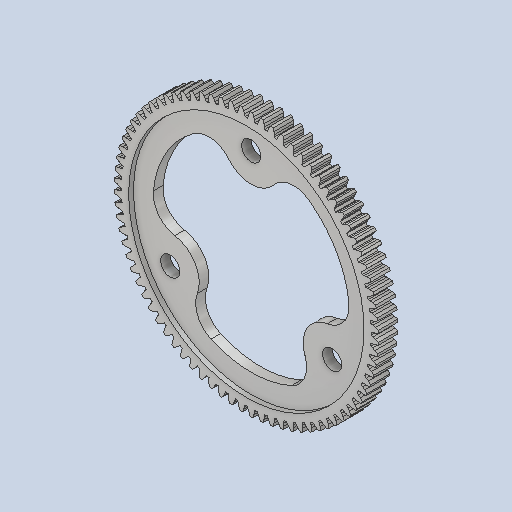
# Autodesk Inventor part: m0.5 80 初段改善
Saved by Autodesk Inventor 2022 (Build 260153000, 153)
## iProperties
Part Number: m0.5 80 初段改善
Material: アセタール樹脂、白
Document SubType Name: Modeling
Designer: user
Density: 1.425 g/cm^3
Appearance: アルミニウム - つや出し
Mass: 1.78935 g
Surface Area: 23.8506 cm^2
Volume: 1.25569 cm^3
Author: user
Autodesk Inventor part; units mm, degrees
(part 1 of 2)
ref_plane "YZ Plane" through (0, 0, 0) normal (1, 0, 0) x (0, 1, 0)
ref_plane "XZ Plane" through (0, 0, 0) normal (0, 1, 0) x (-1, 0, 0)
sketch "スケッチ3" plane through (0, 0, 0) normal (0, 0, 1) x (1, 0, 0)
  circle A0 centre (0, 0) radius 17.5
  circle A1 centre (0, 0) radius 15 construction
  circle A2 centre (-0.0185, 15) radius 3 construction
  arc A3 (1.3802, 16.4422) -> (-1.3922, 16.4412) centre (0, 0) ccw
  arc A4 (15.2271, 6.3549) -> (1.3802, 16.4422) centre (0, 0) ccw
  arc A5 (-1.3922, 16.4412) -> (-15.5317, 5.5691) centre (0, 0) ccw
  arc A6 (-15.7143, -5.031) -> (-7.6771, -14.6052) centre (0, 0) ccw
  arc A7 (-7.6771, -14.6052) -> (3.9215, -16.0272) centre (0, 0) ccw
  arc A8 (3.9215, -16.0272) -> (14.9167, -7.0527) centre (0, 0) ccw
  arc A9 (-15.5317, 5.5691) -> (-15.7143, -5.031) centre (0, 0) ccw
  arc A10 (14.9167, -7.0527) -> (15.2271, 6.3549) centre (0, 0) ccw
  circle A11 centre (-0.0185, 15) radius 1.5
  circle A12 centre (-6.525, 13.5065) radius 1.5
  circle A13 centre (-6.525, 13.5065) radius 3 construction
  circle A14 centre (-11.739, 9.3378) radius 1.5
  circle A15 centre (-11.739, 9.3378) radius 3 construction
  circle A16 centre (-14.628, 3.3197) radius 1.5
  circle A17 centre (-14.628, 3.3197) radius 3 construction
  circle A18 centre (-14.6198, -3.3559) radius 1.5
  circle A19 centre (-14.6198, -3.3559) radius 3 construction
  circle A20 centre (-11.7159, -9.3668) radius 1.5
  circle A21 centre (-11.7159, -9.3668) radius 3 construction
  circle A22 centre (-6.4915, -13.5226) radius 1.5
  circle A23 centre (-6.4915, -13.5226) radius 3 construction
  circle A24 centre (0.0185, -15) radius 1.5
  circle A25 centre (0.0185, -15) radius 3 construction
  circle A26 centre (6.525, -13.5065) radius 1.5
  circle A27 centre (6.525, -13.5065) radius 3 construction
  circle A28 centre (11.739, -9.3378) radius 1.5
  circle A29 centre (11.739, -9.3378) radius 3 construction
  circle A30 centre (14.628, -3.3197) radius 1.5
  circle A31 centre (14.628, -3.3197) radius 3 construction
  circle A32 centre (14.6198, 3.3559) radius 1.5
  circle A33 centre (14.6198, 3.3559) radius 3 construction
  circle A34 centre (11.7159, 9.3668) radius 1.5
  circle A35 centre (11.7159, 9.3668) radius 3 construction
  circle A36 centre (6.4915, 13.5226) radius 1.5
  circle A37 centre (6.4915, 13.5226) radius 3 construction
  circle A38 centre (0, 0) radius 10.5
  point P0 (21.9184, -4.4196)
  dimension "d89" = 30
  dimension "d88" = 35
  dimension "d90" = 6
  dimension "d91" = 33
  dimension "d92" = 3
  dimension "d93" = 360
  dimension "d96" = 21
  constraints: 38 centre point, 20 coincident, 16 point on circle, 60 other
  measures "d88" diameter of A0
  measures "d90" diameter of A2
  measures "d91" diameter of A3
  measures "d92" diameter of A11
  measures "d96" diameter of A38
ref_plane "作業平面1" through (0, 0, 3) normal (0, 0, 1) x (1, 0, 0)
sketch "スケッチ4" plane through (0, 0, 3) normal (0, 0, 1) x (1, 0, 0)
  arc A0 (0.278, 19.6745) -> (0.1896, 19.3741) centre (5.2892, 18.0371) ccw
  arc A1 (0.4118, 20.0451) -> (0.278, 19.6745) centre (6.369, 17.6849) ccw
  arc A2 (0.6052, 20.4911) -> (0.4118, 20.0451) centre (7.4658, 17.2508) ccw
  arc A3 (-1.2665, 19.6357) -> (-1.331, 19.3292) centre (3.8577, 18.3965) ccw
  arc A4 (-1.1622, 20.0156) -> (-1.2665, 19.6357) centre (4.9618, 18.1301) ccw
  arc A5 (-1.0044, 20.4754) -> (-1.1622, 20.0156) centre (6.0894, 17.7834) ccw
  arc A6 (-2.8032, 19.4758) -> (-2.8435, 19.1652) centre (2.4025, 18.6425) ccw
  arc A7 (-2.729, 19.8627) -> (-2.8032, 19.4758) centre (3.5241, 18.4635) ccw
  arc A8 (-2.6078, 20.3335) -> (-2.729, 19.8627) centre (4.6753, 18.2064) ccw
  arc A9 (-4.3226, 19.1958) -> (-4.3384, 18.883) centre (0.9324, 18.7735) ccw
  arc A10 (-4.279, 19.5874) -> (-4.3226, 19.1958) centre (2.0646, 18.6831) ccw
  arc A11 (-4.1951, 20.0662) -> (-4.279, 19.5874) centre (3.2324, 18.517) ccw
  arc A12 (-5.8154, 18.7975) -> (-5.8066, 18.4844) centre (-0.5434, 18.7888) ccw
  arc A13 (-5.8026, 19.1913) -> (-5.8154, 18.7975) centre (0.5924, 18.7875) ccw
  arc A14 (-5.7565, 19.6752) -> (-5.8026, 19.1913) centre (1.7696, 18.7136) ccw
  arc A15 (-7.2723, 18.2833) -> (-7.2389, 17.9719) centre (-2.0159, 18.6882) ccw
  arc A16 (-7.2905, 18.6768) -> (-7.2723, 18.2833) centre (-0.8835, 18.776) ccw
  arc A17 (-7.2825, 19.1629) -> (-7.2905, 18.6768) centre (0.2959, 18.7947) ccw
  arc A18 (-8.6843, 17.6563) -> (-8.6267, 17.3485) centre (-3.476, 18.4724) ccw
  arc A19 (-8.7334, 18.0473) -> (-8.6843, 17.6563) centre (-2.3539, 18.6488) ccw
  arc A20 (-8.7635, 18.5324) -> (-8.7334, 18.0473) centre (-1.1796, 18.76) ccw
  arc A21 (-10.0429, 16.9205) -> (-9.9612, 16.6182) centre (-4.9146, 18.1428) ccw
  arc A22 (-10.122, 17.3041) -> (-10.0429, 16.9205) centre (-3.8099, 18.4067) ccw
  arc A23 (-10.1905, 17.7877) -> (-10.122, 17.3041) centre (-2.6478, 18.6096) ccw
  arc A24 (-11.3395, 16.0804) -> (-11.2344, 15.7854) centre (-6.3229, 17.7012) ccw
  arc A25 (-11.4491, 16.4589) -> (-11.3395, 16.0804) centre (-5.2423, 18.051) ccw
  arc A26 (-11.5547, 16.9334) -> (-11.4491, 16.4589) centre (-4.0998, 18.3445) ccw
  arc A27 (-12.5662, 15.1412) -> (-12.4383, 14.8553) centre (-7.6922, 17.1506) ccw
  arc A28 (-12.7043, 15.5076) -> (-12.5662, 15.1412) centre (-6.6424, 17.5841) ccw
  arc A29 (-12.8477, 15.9746) -> (-12.7043, 15.5076) centre (-5.5264, 17.9663) ccw
  arc A30 (-13.7154, 14.1086) -> (-13.5655, 13.8336) centre (-9.0141, 16.4942) ccw
  arc A31 (-13.8828, 14.4652) -> (-13.7154, 14.1086) centre (-8.0015, 17.0087) ccw
  arc A32 (-14.0614, 14.9173) -> (-13.8828, 14.4652) centre (-6.919, 17.4773) ccw
  arc A33 (-14.7801, 12.989) -> (-14.609, 12.7266) centre (-10.2805, 15.7361) ccw
  arc A34 (-14.975, 13.3314) -> (-14.7801, 12.989) centre (-9.3114, 16.3285) ccw
  arc A35 (-15.1885, 13.7681) -> (-14.975, 13.3314) centre (-8.2689, 16.8806) ccw
  arc A36 (-15.7536, 11.7893) -> (-15.5625, 11.5412) centre (-11.4834, 14.881) ccw
  arc A37 (-15.9748, 12.1154) -> (-15.7536, 11.7893) centre (-10.5638, 15.5476) ccw
  arc A38 (-16.2219, 12.534) -> (-15.9748, 12.1154) centre (-9.5679, 16.1798) ccw
  arc A39 (-16.63, 10.5169) -> (-16.42, 10.2846) centre (-12.6156, 13.9341) ccw
  arc A40 (-16.8761, 10.8246) -> (-16.63, 10.5169) centre (-11.7511, 14.6708) ccw
  arc A41 (-17.1553, 11.2226) -> (-16.8761, 10.8246) centre (-10.8078, 15.3792) ccw
  arc A42 (-17.4039, 9.1797) -> (-17.1763, 8.9646) centre (-13.6699, 12.9014) ccw
  arc A43 (-17.6733, 9.4672) -> (-17.4039, 9.1797) centre (-12.8659, 13.7036) ccw
  arc A44 (-17.9829, 9.842) -> (-17.6733, 9.4672) centre (-11.9812, 14.4838) ccw
  arc A45 (-18.0705, 7.786) -> (-17.8267, 7.5893) centre (-14.64, 11.7891) ccw
  arc A46 (-18.3617, 8.0514) -> (-18.0705, 7.786) centre (-13.9014, 12.6519) ccw
  arc A47 (-18.6997, 8.4007) -> (-18.3617, 8.0514) centre (-13.0806, 13.4991) ccw
  arc A48 (-18.6257, 6.3442) -> (-18.3672, 6.1673) centre (-15.5199, 10.6041) ccw
  arc A49 (-18.9368, 6.5859) -> (-18.6257, 6.3442) centre (-14.8512, 11.5222) ccw
  arc A50 (-19.3011, 6.9077) -> (-18.9368, 6.5859) centre (-14.0994, 12.4312) ccw
  arc A51 (-19.066, 4.8632) -> (-18.7945, 4.7072) centre (-16.304, 9.3537) ccw
  arc A52 (-19.3951, 5.0799) -> (-19.066, 4.8632) centre (-15.7095, 10.3215) ccw
  arc A53 (-19.7836, 5.372) -> (-19.3951, 5.0799) centre (-15.0313, 11.2867) ccw
  arc A54 (-19.3888, 3.3524) -> (-19.1059, 3.2181) centre (-16.9876, 8.0457) ccw
  arc A55 (-19.7339, 3.5425) -> (-19.3888, 3.3524) centre (-16.4708, 9.0571) ccw
  arc A56 (-20.1441, 3.8033) -> (-19.7339, 3.5425) centre (-15.8705, 10.0726) ccw
  arc A57 (-19.592, 1.8208) -> (-19.2995, 1.7091) centre (-17.5665, 6.6881) ccw
  arc A58 (-19.9489, 1.9822) -> (-19.592, 1.8208) centre (-17.1307, 7.7369) ccw
  arc A59 (-20.3804, 2.2111) -> (-19.9489, 1.9822) centre (-16.6119, 8.7963) ccw
  arc A60 (-19.6745, 0.278) -> (-19.3741, 0.1896) centre (-18.0371, 5.2892) ccw
  arc A61 (-20.0429, 0.4109) -> (-19.6745, 0.278) centre (-17.6849, 6.369) ccw
  arc A62 (-20.4911, 0.6052) -> (-20.0429, 0.4109) centre (-17.2508, 7.4658) ccw
  arc A63 (-19.6357, -1.2665) -> (-19.3292, -1.331) centre (-18.3965, 3.8577) ccw
  arc A64 (-20.0156, -1.1622) -> (-19.6357, -1.2665) centre (-18.1301, 4.9618) ccw
  arc A65 (-20.4754, -1.0044) -> (-20.0156, -1.1622) centre (-17.7834, 6.0894) ccw
  arc A66 (-19.4758, -2.8032) -> (-19.1652, -2.8435) centre (-18.6425, 2.4025) ccw
  arc A67 (-19.8604, -2.7295) -> (-19.4758, -2.8032) centre (-18.4635, 3.5241) ccw
  arc A68 (-20.3335, -2.6078) -> (-19.8604, -2.7295) centre (-18.2064, 4.6753) ccw
  arc A69 (-19.1958, -4.3226) -> (-18.883, -4.3384) centre (-18.7735, 0.9324) ccw
  arc A70 (-19.5874, -4.279) -> (-19.1958, -4.3226) centre (-18.6831, 2.0646) ccw
  arc A71 (-20.0662, -4.1951) -> (-19.5874, -4.279) centre (-18.517, 3.2324) ccw
  arc A72 (-18.7975, -5.8154) -> (-18.4844, -5.8066) centre (-18.7888, -0.5434) ccw
  arc A73 (-19.1913, -5.8026) -> (-18.7975, -5.8154) centre (-18.7875, 0.5924) ccw
  arc A74 (-19.6752, -5.7565) -> (-19.1913, -5.8026) centre (-18.7136, 1.7696) ccw
  arc A75 (-18.2833, -7.2723) -> (-17.9719, -7.2389) centre (-18.6882, -2.0159) ccw
  arc A76 (-18.6768, -7.2905) -> (-18.2833, -7.2723) centre (-18.776, -0.8835) ccw
  arc A77 (-19.1629, -7.2825) -> (-18.6768, -7.2905) centre (-18.7947, 0.2959) ccw
  arc A78 (-17.6563, -8.6843) -> (-17.3485, -8.6267) centre (-18.4724, -3.476) ccw
  arc A79 (-18.0473, -8.7334) -> (-17.6563, -8.6843) centre (-18.6488, -2.3539) ccw
  arc A80 (-18.5324, -8.7635) -> (-18.0473, -8.7334) centre (-18.76, -1.1796) ccw
  arc A81 (-16.9205, -10.0429) -> (-16.6182, -9.9612) centre (-18.1428, -4.9146) ccw
  arc A82 (-17.3064, -10.1224) -> (-16.9205, -10.0429) centre (-18.4067, -3.8099) ccw
  arc A83 (-17.7877, -10.1905) -> (-17.3064, -10.1224) centre (-18.6096, -2.6478) ccw
  arc A84 (-16.0804, -11.3395) -> (-15.7854, -11.2344) centre (-17.7012, -6.3229) ccw
  arc A85 (-16.4589, -11.4491) -> (-16.0804, -11.3395) centre (-18.051, -5.2423) ccw
  arc A86 (-16.9334, -11.5547) -> (-16.4589, -11.4491) centre (-18.3445, -4.0998) ccw
  arc A87 (-15.1412, -12.5662) -> (-14.8553, -12.4383) centre (-17.1506, -7.6922) ccw
  arc A88 (-15.5098, -12.7051) -> (-15.1412, -12.5662) centre (-17.5841, -6.6424) ccw
  arc A89 (-15.9746, -12.8477) -> (-15.5098, -12.7051) centre (-17.9663, -5.5264) ccw
  arc A90 (-14.1086, -13.7154) -> (-13.8336, -13.5655) centre (-16.4942, -9.0141) ccw
  arc A91 (-14.4652, -13.8828) -> (-14.1086, -13.7154) centre (-17.0087, -8.0015) ccw
  arc A92 (-14.9173, -14.0614) -> (-14.4652, -13.8828) centre (-17.4773, -6.919) ccw
  arc A93 (-12.989, -14.7801) -> (-12.7266, -14.609) centre (-15.7361, -10.2805) ccw
  arc A94 (-13.3314, -14.975) -> (-12.989, -14.7801) centre (-16.3285, -9.3114) ccw
  arc A95 (-13.7681, -15.1885) -> (-13.3314, -14.975) centre (-16.8806, -8.2689) ccw
  arc A96 (-11.7893, -15.7536) -> (-11.5412, -15.5625) centre (-14.881, -11.4834) ccw
  arc A97 (-12.1154, -15.9748) -> (-11.7893, -15.7536) centre (-15.5476, -10.5638) ccw
  arc A98 (-12.534, -16.2219) -> (-12.1154, -15.9748) centre (-16.1798, -9.5679) ccw
  arc A99 (-10.5169, -16.63) -> (-10.2846, -16.42) centre (-13.9341, -12.6156) ccw
  arc A100 (-10.8246, -16.8761) -> (-10.5169, -16.63) centre (-14.6708, -11.7511) ccw
  arc A101 (-11.2226, -17.1553) -> (-10.8246, -16.8761) centre (-15.3792, -10.8078) ccw
  arc A102 (-9.1797, -17.4039) -> (-8.9646, -17.1763) centre (-12.9014, -13.6699) ccw
  arc A103 (-9.4672, -17.6733) -> (-9.1797, -17.4039) centre (-13.7036, -12.8659) ccw
  arc A104 (-9.842, -17.9829) -> (-9.4672, -17.6733) centre (-14.4838, -11.9812) ccw
  arc A105 (-7.786, -18.0705) -> (-7.5893, -17.8267) centre (-11.7891, -14.64) ccw
  arc A106 (-8.0514, -18.3617) -> (-7.786, -18.0705) centre (-12.6519, -13.9014) ccw
  arc A107 (-8.4007, -18.6997) -> (-8.0514, -18.3617) centre (-13.4991, -13.0806) ccw
  arc A108 (-6.3442, -18.6257) -> (-6.1673, -18.3672) centre (-10.6041, -15.5199) ccw
  arc A109 (-6.5859, -18.9368) -> (-6.3442, -18.6257) centre (-11.5222, -14.8512) ccw
  arc A110 (-6.9077, -19.3011) -> (-6.5859, -18.9368) centre (-12.4312, -14.0994) ccw
  arc A111 (-4.8632, -19.066) -> (-4.7072, -18.7945) centre (-9.3537, -16.304) ccw
  arc A112 (-5.0799, -19.3951) -> (-4.8632, -19.066) centre (-10.3215, -15.7095) ccw
  arc A113 (-5.372, -19.7836) -> (-5.0799, -19.3951) centre (-11.2867, -15.0313) ccw
  arc A114 (-3.3524, -19.3888) -> (-3.2181, -19.1059) centre (-8.0457, -16.9876) ccw
  arc A115 (-3.5425, -19.7339) -> (-3.3524, -19.3888) centre (-9.0571, -16.4708) ccw
  arc A116 (-3.8033, -20.1441) -> (-3.5425, -19.7339) centre (-10.0726, -15.8705) ccw
  arc A117 (-1.8197, -19.5895) -> (-1.7091, -19.2995) centre (-6.6881, -17.5665) ccw
  arc A118 (-1.9832, -19.951) -> (-1.8197, -19.5895) centre (-7.7369, -17.1307) ccw
  arc A119 (-2.2111, -20.3804) -> (-1.9832, -19.951) centre (-8.7963, -16.6119) ccw
  arc A120 (-0.278, -19.6745) -> (-0.1896, -19.3741) centre (-5.2892, -18.0371) ccw
  arc A121 (-0.4109, -20.0429) -> (-0.278, -19.6745) centre (-6.369, -17.6849) ccw
  arc A122 (-0.6052, -20.4911) -> (-0.4109, -20.0429) centre (-7.4658, -17.2508) ccw
  arc A123 (1.2665, -19.6357) -> (1.331, -19.3292) centre (-3.8577, -18.3965) ccw
  arc A124 (1.1622, -20.0156) -> (1.2665, -19.6357) centre (-4.9618, -18.1301) ccw
  arc A125 (1.0044, -20.4754) -> (1.1622, -20.0156) centre (-6.0894, -17.7834) ccw
  arc A126 (2.8032, -19.4758) -> (2.8435, -19.1652) centre (-2.4025, -18.6425) ccw
  arc A127 (2.729, -19.8627) -> (2.8032, -19.4758) centre (-3.5241, -18.4635) ccw
  arc A128 (2.6078, -20.3335) -> (2.729, -19.8627) centre (-4.6753, -18.2064) ccw
  arc A129 (4.3226, -19.1958) -> (4.3384, -18.883) centre (-0.9324, -18.7735) ccw
  arc A130 (4.279, -19.5874) -> (4.3226, -19.1958) centre (-2.0646, -18.6831) ccw
  arc A131 (4.1951, -20.0662) -> (4.279, -19.5874) centre (-3.2324, -18.517) ccw
  arc A132 (5.8154, -18.7975) -> (5.8066, -18.4844) centre (0.5434, -18.7888) ccw
  arc A133 (5.8026, -19.1913) -> (5.8154, -18.7975) centre (-0.5924, -18.7875) ccw
  arc A134 (5.7565, -19.6752) -> (5.8026, -19.1913) centre (-1.7696, -18.7136) ccw
  arc A135 (7.2723, -18.2833) -> (7.2389, -17.9719) centre (2.0159, -18.6882) ccw
  arc A136 (7.2905, -18.6768) -> (7.2723, -18.2833) centre (0.8835, -18.776) ccw
  arc A137 (7.2825, -19.1629) -> (7.2905, -18.6768) centre (-0.2959, -18.7947) ccw
  arc A138 (8.6843, -17.6563) -> (8.6267, -17.3485) centre (3.476, -18.4724) ccw
  arc A139 (8.7334, -18.0473) -> (8.6843, -17.6563) centre (2.3539, -18.6488) ccw
  arc A140 (8.7635, -18.5324) -> (8.7334, -18.0473) centre (1.1796, -18.76) ccw
  arc A141 (10.0429, -16.9205) -> (9.9612, -16.6182) centre (4.9146, -18.1428) ccw
  arc A142 (10.1224, -17.3064) -> (10.0429, -16.9205) centre (3.8099, -18.4067) ccw
  arc A143 (10.1905, -17.7877) -> (10.1224, -17.3064) centre (2.6478, -18.6096) ccw
  arc A144 (11.3395, -16.0804) -> (11.2344, -15.7854) centre (6.3229, -17.7012) ccw
  arc A145 (11.4485, -16.4566) -> (11.3395, -16.0804) centre (5.2423, -18.051) ccw
  arc A146 (11.5547, -16.9334) -> (11.4485, -16.4566) centre (4.0998, -18.3445) ccw
  arc A147 (12.5662, -15.1412) -> (12.4383, -14.8553) centre (7.6922, -17.1506) ccw
  arc A148 (12.7051, -15.5098) -> (12.5662, -15.1412) centre (6.6424, -17.5841) ccw
  arc A149 (12.8477, -15.9746) -> (12.7051, -15.5098) centre (5.5264, -17.9663) ccw
  arc A150 (13.7154, -14.1086) -> (13.5655, -13.8336) centre (9.0141, -16.4942) ccw
  arc A151 (13.8828, -14.4652) -> (13.7154, -14.1086) centre (8.0015, -17.0087) ccw
  arc A152 (14.0614, -14.9173) -> (13.8828, -14.4652) centre (6.919, -17.4773) ccw
  arc A153 (14.7801, -12.989) -> (14.609, -12.7266) centre (10.2805, -15.7361) ccw
  arc A154 (14.975, -13.3314) -> (14.7801, -12.989) centre (9.3114, -16.3285) ccw
  arc A155 (15.1885, -13.7681) -> (14.975, -13.3314) centre (8.2689, -16.8806) ccw
  arc A156 (15.7536, -11.7893) -> (15.5625, -11.5412) centre (11.4834, -14.881) ccw
  arc A157 (15.9748, -12.1154) -> (15.7536, -11.7893) centre (10.5638, -15.5476) ccw
  arc A158 (16.2219, -12.534) -> (15.9748, -12.1154) centre (9.5679, -16.1798) ccw
  arc A159 (16.63, -10.5169) -> (16.42, -10.2846) centre (12.6156, -13.9341) ccw
  arc A160 (16.8761, -10.8246) -> (16.63, -10.5169) centre (11.7511, -14.6708) ccw
  arc A161 (17.1553, -11.2226) -> (16.8761, -10.8246) centre (10.8078, -15.3792) ccw
  arc A162 (17.4039, -9.1797) -> (17.1763, -8.9646) centre (13.6699, -12.9014) ccw
  arc A163 (17.6718, -9.4654) -> (17.4039, -9.1797) centre (12.8659, -13.7036) ccw
  arc A164 (17.9829, -9.842) -> (17.6718, -9.4654) centre (11.9812, -14.4838) ccw
  arc A165 (18.0705, -7.786) -> (17.8267, -7.5893) centre (14.64, -11.7891) ccw
  arc A166 (18.36, -8.0497) -> (18.0705, -7.786) centre (13.9014, -12.6519) ccw
  arc A167 (18.6997, -8.4007) -> (18.36, -8.0497) centre (13.0806, -13.4991) ccw
  arc A168 (18.6257, -6.3442) -> (18.3672, -6.1673) centre (15.5199, -10.6041) ccw
  arc A169 (18.9349, -6.5844) -> (18.6257, -6.3442) centre (14.8512, -11.5222) ccw
  arc A170 (19.3011, -6.9077) -> (18.9349, -6.5844) centre (14.0994, -12.4312) ccw
  arc A171 (19.066, -4.8632) -> (18.7945, -4.7072) centre (16.304, -9.3537) ccw
  arc A172 (19.3932, -5.0785) -> (19.066, -4.8632) centre (15.7095, -10.3215) ccw
  arc A173 (19.7836, -5.372) -> (19.3932, -5.0785) centre (15.0313, -11.2867) ccw
  arc A174 (19.3888, -3.3524) -> (19.1059, -3.2181) centre (16.9876, -8.0457) ccw
  arc A175 (19.7318, -3.5413) -> (19.3888, -3.3524) centre (16.4708, -9.0571) ccw
  arc A176 (20.1441, -3.8033) -> (19.7318, -3.5413) centre (15.8705, -10.0726) ccw
  arc A177 (19.592, -1.8208) -> (19.2995, -1.7091) centre (17.5665, -6.6881) ccw
  arc A178 (19.9489, -1.9822) -> (19.592, -1.8208) centre (17.1307, -7.7369) ccw
  arc A179 (20.3804, -2.2111) -> (19.9489, -1.9822) centre (16.6119, -8.7963) ccw
  arc A180 (19.6745, -0.278) -> (19.3741, -0.1896) centre (18.0371, -5.2892) ccw
  arc A181 (20.0451, -0.4118) -> (19.6745, -0.278) centre (17.6849, -6.369) ccw
  arc A182 (20.4911, -0.6052) -> (20.0451, -0.4118) centre (17.2508, -7.4658) ccw
  arc A183 (19.6357, 1.2665) -> (19.3292, 1.331) centre (18.3965, -3.8577) ccw
  arc A184 (20.0156, 1.1622) -> (19.6357, 1.2665) centre (18.1301, -4.9618) ccw
  arc A185 (20.4754, 1.0044) -> (20.0156, 1.1622) centre (17.7834, -6.0894) ccw
  arc A186 (19.4758, 2.8032) -> (19.1652, 2.8435) centre (18.6425, -2.4025) ccw
  arc A187 (19.8627, 2.729) -> (19.4758, 2.8032) centre (18.4635, -3.5241) ccw
  arc A188 (20.3335, 2.6078) -> (19.8627, 2.729) centre (18.2064, -4.6753) ccw
  arc A189 (19.1958, 4.3226) -> (18.883, 4.3384) centre (18.7735, -0.9324) ccw
  arc A190 (19.585, 4.2793) -> (19.1958, 4.3226) centre (18.6831, -2.0646) ccw
  arc A191 (20.0662, 4.1951) -> (19.585, 4.2793) centre (18.517, -3.2324) ccw
  arc A192 (18.7975, 5.8154) -> (18.4844, 5.8066) centre (18.7888, 0.5434) ccw
  arc A193 (19.1889, 5.8028) -> (18.7975, 5.8154) centre (18.7875, -0.5924) ccw
  arc A194 (19.6752, 5.7565) -> (19.1889, 5.8028) centre (18.7136, -1.7696) ccw
  arc A195 (18.2833, 7.2723) -> (17.9719, 7.2389) centre (18.6882, 2.0159) ccw
  arc A196 (18.6768, 7.2905) -> (18.2833, 7.2723) centre (18.776, 0.8835) ccw
  arc A197 (19.1629, 7.2825) -> (18.6768, 7.2905) centre (18.7947, -0.2959) ccw
  arc A198 (17.6563, 8.6843) -> (17.3485, 8.6267) centre (18.4724, 3.476) ccw
  arc A199 (18.0473, 8.7334) -> (17.6563, 8.6843) centre (18.6488, 2.3539) ccw
  arc A200 (18.5324, 8.7635) -> (18.0473, 8.7334) centre (18.76, 1.1796) ccw
  arc A201 (16.9205, 10.0429) -> (16.6182, 9.9612) centre (18.1428, 4.9146) ccw
  arc A202 (17.3064, 10.1224) -> (16.9205, 10.0429) centre (18.4067, 3.8099) ccw
  arc A203 (17.7877, 10.1905) -> (17.3064, 10.1224) centre (18.6096, 2.6478) ccw
  arc A204 (16.0804, 11.3395) -> (15.7854, 11.2344) centre (17.7012, 6.3229) ccw
  arc A205 (16.4589, 11.4491) -> (16.0804, 11.3395) centre (18.051, 5.2423) ccw
  arc A206 (16.9334, 11.5547) -> (16.4589, 11.4491) centre (18.3445, 4.0998) ccw
  arc A207 (15.1412, 12.5662) -> (14.8553, 12.4383) centre (17.1506, 7.6922) ccw
  arc A208 (15.5098, 12.7051) -> (15.1412, 12.5662) centre (17.5841, 6.6424) ccw
  arc A209 (15.9746, 12.8477) -> (15.5098, 12.7051) centre (17.9663, 5.5264) ccw
  arc A210 (14.1086, 13.7154) -> (13.8336, 13.5655) centre (16.4942, 9.0141) ccw
  arc A211 (14.4652, 13.8828) -> (14.1086, 13.7154) centre (17.0087, 8.0015) ccw
  arc A212 (14.9173, 14.0614) -> (14.4652, 13.8828) centre (17.4773, 6.919) ccw
  arc A213 (12.989, 14.7801) -> (12.7266, 14.609) centre (15.7361, 10.2805) ccw
  arc A214 (13.3314, 14.975) -> (12.989, 14.7801) centre (16.3285, 9.3114) ccw
  arc A215 (13.7681, 15.1885) -> (13.3314, 14.975) centre (16.8806, 8.2689) ccw
  arc A216 (11.7893, 15.7536) -> (11.5412, 15.5625) centre (14.881, 11.4834) ccw
  arc A217 (12.1154, 15.9748) -> (11.7893, 15.7536) centre (15.5476, 10.5638) ccw
  arc A218 (12.534, 16.2219) -> (12.1154, 15.9748) centre (16.1798, 9.5679) ccw
  arc A219 (10.5169, 16.63) -> (10.2846, 16.42) centre (13.9341, 12.6156) ccw
  arc A220 (10.8246, 16.8761) -> (10.5169, 16.63) centre (14.6708, 11.7511) ccw
  arc A221 (11.2226, 17.1553) -> (10.8246, 16.8761) centre (15.3792, 10.8078) ccw
  arc A222 (9.1797, 17.4039) -> (8.9646, 17.1763) centre (12.9014, 13.6699) ccw
  arc A223 (9.4672, 17.6733) -> (9.1797, 17.4039) centre (13.7036, 12.8659) ccw
  arc A224 (9.842, 17.9829) -> (9.4672, 17.6733) centre (14.4838, 11.9812) ccw
  arc A225 (7.786, 18.0705) -> (7.5893, 17.8267) centre (11.7891, 14.64) ccw
  arc A226 (8.0514, 18.3617) -> (7.786, 18.0705) centre (12.6519, 13.9014) ccw
  arc A227 (8.4007, 18.6997) -> (8.0514, 18.3617) centre (13.4991, 13.0806) ccw
  arc A228 (6.3442, 18.6257) -> (6.1673, 18.3672) centre (10.6041, 15.5199) ccw
  arc A229 (6.5859, 18.9368) -> (6.3442, 18.6257) centre (11.5222, 14.8512) ccw
  arc A230 (6.9077, 19.3011) -> (6.5859, 18.9368) centre (12.4312, 14.0994) ccw
  arc A231 (4.8632, 19.066) -> (4.7072, 18.7945) centre (9.3537, 16.304) ccw
  arc A232 (5.0799, 19.3951) -> (4.8632, 19.066) centre (10.3215, 15.7095) ccw
  arc A233 (5.372, 19.7836) -> (5.0799, 19.3951) centre (11.2867, 15.0313) ccw
  arc A234 (3.3524, 19.3888) -> (3.2181, 19.1059) centre (8.0457, 16.9876) ccw
  arc A235 (3.5425, 19.7339) -> (3.3524, 19.3888) centre (9.0571, 16.4708) ccw
  arc A236 (3.8033, 20.1441) -> (3.5425, 19.7339) centre (10.0726, 15.8705) ccw
  arc A237 (1.8208, 19.592) -> (1.7091, 19.2995) centre (6.6881, 17.5665) ccw
  arc A238 (1.9832, 19.951) -> (1.8208, 19.592) centre (7.7369, 17.1307) ccw
  arc A239 (2.2111, 20.3804) -> (1.9832, 19.951) centre (8.7963, 16.6119) ccw
  arc A240 (-0.1896, 19.3741) -> (-0.278, 19.6745) centre (-5.2892, 18.0371) ccw
  arc A241 (-0.278, 19.6745) -> (-0.4118, 20.0451) centre (-6.369, 17.6849) ccw
  arc A242 (-0.4118, 20.0451) -> (-0.6052, 20.4911) centre (-7.4658, 17.2508) ccw
  arc A243 (-1.7091, 19.2995) -> (-1.8208, 19.592) centre (-6.6881, 17.5665) ccw
  arc A244 (-1.8208, 19.592) -> (-1.9832, 19.951) centre (-7.7369, 17.1307) ccw
  arc A245 (-1.9832, 19.951) -> (-2.2111, 20.3804) centre (-8.7963, 16.6119) ccw
  arc A246 (-3.2181, 19.1059) -> (-3.3524, 19.3888) centre (-8.0457, 16.9876) ccw
  arc A247 (-3.3524, 19.3888) -> (-3.5425, 19.7339) centre (-9.0571, 16.4708) ccw
  arc A248 (-3.5425, 19.7339) -> (-3.8033, 20.1441) centre (-10.0726, 15.8705) ccw
  arc A249 (-4.7072, 18.7945) -> (-4.8632, 19.066) centre (-9.3537, 16.304) ccw
  arc A250 (-4.8632, 19.066) -> (-5.0799, 19.3951) centre (-10.3215, 15.7095) ccw
  arc A251 (-5.0799, 19.3951) -> (-5.372, 19.7836) centre (-11.2867, 15.0313) ccw
  arc A252 (-6.1673, 18.3672) -> (-6.3442, 18.6257) centre (-10.6041, 15.5199) ccw
  arc A253 (-6.3442, 18.6257) -> (-6.5859, 18.9368) centre (-11.5222, 14.8512) ccw
  arc A254 (-6.5859, 18.9368) -> (-6.9077, 19.3011) centre (-12.4312, 14.0994) ccw
  arc A255 (-7.5893, 17.8267) -> (-7.786, 18.0705) centre (-11.7891, 14.64) ccw
  arc A256 (-7.786, 18.0705) -> (-8.0514, 18.3617) centre (-12.6519, 13.9014) ccw
  arc A257 (-8.0514, 18.3617) -> (-8.4007, 18.6997) centre (-13.4991, 13.0806) ccw
  arc A258 (-8.9646, 17.1763) -> (-9.1797, 17.4039) centre (-12.9014, 13.6699) ccw
  arc A259 (-9.1797, 17.4039) -> (-9.4672, 17.6733) centre (-13.7036, 12.8659) ccw
  arc A260 (-9.4672, 17.6733) -> (-9.842, 17.9829) centre (-14.4838, 11.9812) ccw
  arc A261 (-10.2846, 16.42) -> (-10.5169, 16.63) centre (-13.9341, 12.6156) ccw
  arc A262 (-10.5169, 16.63) -> (-10.8246, 16.8761) centre (-14.6708, 11.7511) ccw
  arc A263 (-10.8246, 16.8761) -> (-11.2226, 17.1553) centre (-15.3792, 10.8078) ccw
  arc A264 (-11.5412, 15.5625) -> (-11.7893, 15.7536) centre (-14.881, 11.4834) ccw
  arc A265 (-11.7893, 15.7536) -> (-12.1154, 15.9748) centre (-15.5476, 10.5638) ccw
  arc A266 (-12.1154, 15.9748) -> (-12.534, 16.2219) centre (-16.1798, 9.5679) ccw
  arc A267 (-12.7266, 14.609) -> (-12.989, 14.7801) centre (-15.7361, 10.2805) ccw
  arc A268 (-12.989, 14.7801) -> (-13.3314, 14.975) centre (-16.3285, 9.3114) ccw
  arc A269 (-13.3314, 14.975) -> (-13.7681, 15.1885) centre (-16.8806, 8.2689) ccw
  arc A270 (-13.8336, 13.5655) -> (-14.1086, 13.7154) centre (-16.4942, 9.0141) ccw
  arc A271 (-14.1086, 13.7154) -> (-14.4652, 13.8828) centre (-17.0087, 8.0015) ccw
  arc A272 (-14.4652, 13.8828) -> (-14.9173, 14.0614) centre (-17.4773, 6.919) ccw
  arc A273 (-14.8553, 12.4383) -> (-15.1412, 12.5662) centre (-17.1506, 7.6922) ccw
  arc A274 (-15.1412, 12.5662) -> (-15.5098, 12.7051) centre (-17.5841, 6.6424) ccw
  arc A275 (-15.5098, 12.7051) -> (-15.9746, 12.8477) centre (-17.9663, 5.5264) ccw
  arc A276 (-15.7854, 11.2344) -> (-16.0804, 11.3395) centre (-17.7012, 6.3229) ccw
  arc A277 (-16.0804, 11.3395) -> (-16.4589, 11.4491) centre (-18.051, 5.2423) ccw
  arc A278 (-16.4589, 11.4491) -> (-16.9334, 11.5547) centre (-18.3445, 4.0998) ccw
  arc A279 (-16.6182, 9.9612) -> (-16.9205, 10.0429) centre (-18.1428, 4.9146) ccw
  arc A280 (-16.9205, 10.0429) -> (-17.3064, 10.1224) centre (-18.4067, 3.8099) ccw
  arc A281 (-17.3064, 10.1224) -> (-17.7877, 10.1905) centre (-18.6096, 2.6478) ccw
  arc A282 (-17.3485, 8.6267) -> (-17.6563, 8.6843) centre (-18.4724, 3.476) ccw
  arc A283 (-17.6563, 8.6843) -> (-18.0473, 8.7334) centre (-18.6488, 2.3539) ccw
  arc A284 (-18.0473, 8.7334) -> (-18.5324, 8.7635) centre (-18.76, 1.1796) ccw
  arc A285 (-17.9719, 7.2389) -> (-18.2833, 7.2723) centre (-18.6882, 2.0159) ccw
  arc A286 (-18.2833, 7.2723) -> (-18.6768, 7.2905) centre (-18.776, 0.8835) ccw
  arc A287 (-18.6768, 7.2905) -> (-19.1629, 7.2825) centre (-18.7947, -0.2959) ccw
  arc A288 (-18.4844, 5.8066) -> (-18.7975, 5.8154) centre (-18.7888, 0.5434) ccw
  arc A289 (-18.7975, 5.8154) -> (-19.1913, 5.8026) centre (-18.7875, -0.5924) ccw
  arc A290 (-19.1913, 5.8026) -> (-19.6752, 5.7565) centre (-18.7136, -1.7696) ccw
  arc A291 (-18.883, 4.3384) -> (-19.1958, 4.3226) centre (-18.7735, -0.9324) ccw
  arc A292 (-19.1958, 4.3226) -> (-19.5874, 4.279) centre (-18.6831, -2.0646) ccw
  arc A293 (-19.5874, 4.279) -> (-20.0662, 4.1951) centre (-18.517, -3.2324) ccw
  arc A294 (-19.1652, 2.8435) -> (-19.4758, 2.8032) centre (-18.6425, -2.4025) ccw
  arc A295 (-19.4758, 2.8032) -> (-19.8627, 2.729) centre (-18.4635, -3.5241) ccw
  arc A296 (-19.8627, 2.729) -> (-20.3335, 2.6078) centre (-18.2064, -4.6753) ccw
  arc A297 (-19.3292, 1.331) -> (-19.6357, 1.2665) centre (-18.3965, -3.8577) ccw
  arc A298 (-19.6357, 1.2665) -> (-20.0156, 1.1622) centre (-18.1301, -4.9618) ccw
  arc A299 (-20.0156, 1.1622) -> (-20.4754, 1.0044) centre (-17.7834, -6.0894) ccw
  arc A300 (-19.3741, -0.1896) -> (-19.6745, -0.278) centre (-18.0371, -5.2892) ccw
  arc A301 (-19.6745, -0.278) -> (-20.0429, -0.4109) centre (-17.6849, -6.369) ccw
  arc A302 (-20.0429, -0.4109) -> (-20.4911, -0.6052) centre (-17.2508, -7.4658) ccw
  arc A303 (-19.2995, -1.7091) -> (-19.592, -1.8208) centre (-17.5665, -6.6881) ccw
  arc A304 (-19.592, -1.8208) -> (-19.951, -1.9832) centre (-17.1307, -7.7369) ccw
  arc A305 (-19.951, -1.9832) -> (-20.3804, -2.2111) centre (-16.6119, -8.7963) ccw
  arc A306 (-19.1059, -3.2181) -> (-19.3888, -3.3524) centre (-16.9876, -8.0457) ccw
  arc A307 (-19.3888, -3.3524) -> (-19.7318, -3.5413) centre (-16.4708, -9.0571) ccw
  arc A308 (-19.7318, -3.5413) -> (-20.1441, -3.8033) centre (-15.8705, -10.0726) ccw
  arc A309 (-18.7945, -4.7072) -> (-19.066, -4.8632) centre (-16.304, -9.3537) ccw
  arc A310 (-19.066, -4.8632) -> (-19.3951, -5.0799) centre (-15.7095, -10.3215) ccw
  arc A311 (-19.3951, -5.0799) -> (-19.7836, -5.372) centre (-15.0313, -11.2867) ccw
  arc A312 (-18.3672, -6.1673) -> (-18.6257, -6.3442) centre (-15.5199, -10.6041) ccw
  arc A313 (-18.6257, -6.3442) -> (-18.9368, -6.5859) centre (-14.8512, -11.5222) ccw
  arc A314 (-18.9368, -6.5859) -> (-19.3011, -6.9077) centre (-14.0994, -12.4312) ccw
  arc A315 (-17.8267, -7.5893) -> (-18.0705, -7.786) centre (-14.64, -11.7891) ccw
  arc A316 (-18.0705, -7.786) -> (-18.3617, -8.0514) centre (-13.9014, -12.6519) ccw
  arc A317 (-18.3617, -8.0514) -> (-18.6997, -8.4007) centre (-13.0806, -13.4991) ccw
  arc A318 (-17.1763, -8.9646) -> (-17.4039, -9.1797) centre (-13.6699, -12.9014) ccw
  arc A319 (-17.4039, -9.1797) -> (-17.6733, -9.4672) centre (-12.8659, -13.7036) ccw
  arc A320 (-17.6733, -9.4672) -> (-17.9829, -9.842) centre (-11.9812, -14.4838) ccw
  arc A321 (-16.42, -10.2846) -> (-16.63, -10.5169) centre (-12.6156, -13.9341) ccw
  arc A322 (-16.63, -10.5169) -> (-16.8761, -10.8246) centre (-11.7511, -14.6708) ccw
  arc A323 (-16.8761, -10.8246) -> (-17.1553, -11.2226) centre (-10.8078, -15.3792) ccw
  arc A324 (-15.5625, -11.5412) -> (-15.7536, -11.7893) centre (-11.4834, -14.881) ccw
  arc A325 (-15.7536, -11.7893) -> (-15.9748, -12.1154) centre (-10.5638, -15.5476) ccw
  arc A326 (-15.9748, -12.1154) -> (-16.2219, -12.534) centre (-9.5679, -16.1798) ccw
  arc A327 (-14.609, -12.7266) -> (-14.7801, -12.989) centre (-10.2805, -15.7361) ccw
  arc A328 (-14.7801, -12.989) -> (-14.975, -13.3314) centre (-9.3114, -16.3285) ccw
  arc A329 (-14.975, -13.3314) -> (-15.1885, -13.7681) centre (-8.2689, -16.8806) ccw
  arc A330 (-13.5655, -13.8336) -> (-13.7154, -14.1086) centre (-9.0141, -16.4942) ccw
  arc A331 (-13.7154, -14.1086) -> (-13.8828, -14.4652) centre (-8.0015, -17.0087) ccw
  arc A332 (-13.8828, -14.4652) -> (-14.0614, -14.9173) centre (-6.919, -17.4773) ccw
  arc A333 (-12.4383, -14.8553) -> (-12.5662, -15.1412) centre (-7.6922, -17.1506) ccw
  arc A334 (-12.5662, -15.1412) -> (-12.7051, -15.5098) centre (-6.6424, -17.5841) ccw
  arc A335 (-12.7051, -15.5098) -> (-12.8477, -15.9746) centre (-5.5264, -17.9663) ccw
  arc A336 (-11.2344, -15.7854) -> (-11.3395, -16.0804) centre (-6.3229, -17.7012) ccw
  arc A337 (-11.3395, -16.0804) -> (-11.4491, -16.4589) centre (-5.2423, -18.051) ccw
  arc A338 (-11.4491, -16.4589) -> (-11.5547, -16.9334) centre (-4.0998, -18.3445) ccw
  arc A339 (-9.9612, -16.6182) -> (-10.0429, -16.9205) centre (-4.9146, -18.1428) ccw
  arc A340 (-10.0429, -16.9205) -> (-10.1224, -17.3064) centre (-3.8099, -18.4067) ccw
  arc A341 (-10.1224, -17.3064) -> (-10.1905, -17.7877) centre (-2.6478, -18.6096) ccw
  arc A342 (-8.6267, -17.3485) -> (-8.6839, -17.6536) centre (-3.476, -18.4724) ccw
  arc A343 (-8.6839, -17.6536) -> (-8.7334, -18.0473) centre (-2.3539, -18.6488) ccw
  arc A344 (-8.7334, -18.0473) -> (-8.7635, -18.5324) centre (-1.1796, -18.76) ccw
  arc A345 (-7.2389, -17.9719) -> (-7.272, -18.2805) centre (-2.0159, -18.6882) ccw
  arc A346 (-7.272, -18.2805) -> (-7.2905, -18.6768) centre (-0.8835, -18.776) ccw
  arc A347 (-7.2905, -18.6768) -> (-7.2825, -19.1629) centre (0.2959, -18.7947) ccw
  arc A348 (-5.8066, -18.4844) -> (-5.8154, -18.7975) centre (-0.5434, -18.7888) ccw
  arc A349 (-5.8154, -18.7975) -> (-5.8026, -19.1913) centre (0.5924, -18.7875) ccw
  arc A350 (-5.8026, -19.1913) -> (-5.7565, -19.6752) centre (1.7696, -18.7136) ccw
  arc A351 (-4.3384, -18.883) -> (-4.3226, -19.1958) centre (0.9324, -18.7735) ccw
  arc A352 (-4.3226, -19.1958) -> (-4.279, -19.5874) centre (2.0646, -18.6831) ccw
  arc A353 (-4.279, -19.5874) -> (-4.1951, -20.0662) centre (3.2324, -18.517) ccw
  arc A354 (-2.8435, -19.1652) -> (-2.8032, -19.4758) centre (2.4025, -18.6425) ccw
  arc A355 (-2.8032, -19.4758) -> (-2.729, -19.8627) centre (3.5241, -18.4635) ccw
  arc A356 (-2.729, -19.8627) -> (-2.6078, -20.3335) centre (4.6753, -18.2064) ccw
  arc A357 (-1.331, -19.3292) -> (-1.2665, -19.6357) centre (3.8577, -18.3965) ccw
  arc A358 (-1.2665, -19.6357) -> (-1.1622, -20.0156) centre (4.9618, -18.1301) ccw
  arc A359 (-1.1622, -20.0156) -> (-1.0044, -20.4754) centre (6.0894, -17.7834) ccw
  arc A360 (0.1896, -19.3741) -> (0.278, -19.6745) centre (5.2892, -18.0371) ccw
  arc A361 (0.278, -19.6745) -> (0.4118, -20.0451) centre (6.369, -17.6849) ccw
  arc A362 (0.4118, -20.0451) -> (0.6052, -20.4911) centre (7.4658, -17.2508) ccw
  arc A363 (1.7091, -19.2995) -> (1.8208, -19.592) centre (6.6881, -17.5665) ccw
  arc A364 (1.8208, -19.592) -> (1.9832, -19.951) centre (7.7369, -17.1307) ccw
  arc A365 (1.9832, -19.951) -> (2.2111, -20.3804) centre (8.7963, -16.6119) ccw
  arc A366 (3.2181, -19.1059) -> (3.3524, -19.3888) centre (8.0457, -16.9876) ccw
  arc A367 (3.3524, -19.3888) -> (3.5425, -19.7339) centre (9.0571, -16.4708) ccw
  arc A368 (3.5425, -19.7339) -> (3.8033, -20.1441) centre (10.0726, -15.8705) ccw
  arc A369 (4.7072, -18.7945) -> (4.8618, -19.0636) centre (9.3537, -16.304) ccw
  arc A370 (4.8618, -19.0636) -> (5.0799, -19.3951) centre (10.3215, -15.7095) ccw
  arc A371 (5.0799, -19.3951) -> (5.372, -19.7836) centre (11.2867, -15.0313) ccw
  arc A372 (6.1673, -18.3672) -> (6.3442, -18.6257) centre (10.6041, -15.5199) ccw
  arc A373 (6.3442, -18.6257) -> (6.5844, -18.9349) centre (11.5222, -14.8512) ccw
  arc A374 (6.5844, -18.9349) -> (6.9077, -19.3011) centre (12.4312, -14.0994) ccw
  arc A375 (7.5893, -17.8267) -> (7.7842, -18.0684) centre (11.7891, -14.64) ccw
  arc A376 (7.7842, -18.0684) -> (8.0514, -18.3617) centre (12.6519, -13.9014) ccw
  arc A377 (8.0514, -18.3617) -> (8.4007, -18.6997) centre (13.4991, -13.0806) ccw
  arc A378 (8.9646, -17.1763) -> (9.1797, -17.4039) centre (12.9014, -13.6699) ccw
  arc A379 (9.1797, -17.4039) -> (9.4672, -17.6733) centre (13.7036, -12.8659) ccw
  arc A380 (9.4672, -17.6733) -> (9.842, -17.9829) centre (14.4838, -11.9812) ccw
  arc A381 (10.2846, -16.42) -> (10.5169, -16.63) centre (13.9341, -12.6156) ccw
  arc A382 (10.5169, -16.63) -> (10.8246, -16.8761) centre (14.6708, -11.7511) ccw
  arc A383 (10.8246, -16.8761) -> (11.2226, -17.1553) centre (15.3792, -10.8078) ccw
  arc A384 (11.5412, -15.5625) -> (11.7893, -15.7536) centre (14.881, -11.4834) ccw
  arc A385 (11.7893, -15.7536) -> (12.1154, -15.9748) centre (15.5476, -10.5638) ccw
  arc A386 (12.1154, -15.9748) -> (12.534, -16.2219) centre (16.1798, -9.5679) ccw
  arc A387 (12.7266, -14.609) -> (12.989, -14.7801) centre (15.7361, -10.2805) ccw
  arc A388 (12.989, -14.7801) -> (13.3314, -14.975) centre (16.3285, -9.3114) ccw
  arc A389 (13.3314, -14.975) -> (13.7681, -15.1885) centre (16.8806, -8.2689) ccw
  arc A390 (13.8336, -13.5655) -> (14.1086, -13.7154) centre (16.4942, -9.0141) ccw
  arc A391 (14.1086, -13.7154) -> (14.4652, -13.8828) centre (17.0087, -8.0015) ccw
  arc A392 (14.4652, -13.8828) -> (14.9173, -14.0614) centre (17.4773, -6.919) ccw
  arc A393 (14.8553, -12.4383) -> (15.1412, -12.5662) centre (17.1506, -7.6922) ccw
  arc A394 (15.1412, -12.5662) -> (15.5098, -12.7051) centre (17.5841, -6.6424) ccw
  arc A395 (15.5098, -12.7051) -> (15.9746, -12.8477) centre (17.9663, -5.5264) ccw
  arc A396 (15.7854, -11.2344) -> (16.0804, -11.3395) centre (17.7012, -6.3229) ccw
  arc A397 (16.0804, -11.3395) -> (16.4566, -11.4485) centre (18.051, -5.2423) ccw
  arc A398 (16.4566, -11.4485) -> (16.9334, -11.5547) centre (18.3445, -4.0998) ccw
  arc A399 (16.6182, -9.9612) -> (16.9205, -10.0429) centre (18.1428, -4.9146) ccw
  arc A400 (16.9205, -10.0429) -> (17.3064, -10.1224) centre (18.4067, -3.8099) ccw
  arc A401 (17.3064, -10.1224) -> (17.7877, -10.1905) centre (18.6096, -2.6478) ccw
  arc A402 (17.3485, -8.6267) -> (17.6536, -8.6839) centre (18.4724, -3.476) ccw
  arc A403 (17.6536, -8.6839) -> (18.0473, -8.7334) centre (18.6488, -2.3539) ccw
  arc A404 (18.0473, -8.7334) -> (18.5324, -8.7635) centre (18.76, -1.1796) ccw
  arc A405 (17.9719, -7.2389) -> (18.2833, -7.2723) centre (18.6882, -2.0159) ccw
  arc A406 (18.2833, -7.2723) -> (18.6768, -7.2905) centre (18.776, -0.8835) ccw
  arc A407 (18.6768, -7.2905) -> (19.1629, -7.2825) centre (18.7947, 0.2959) ccw
  arc A408 (18.4844, -5.8066) -> (18.7975, -5.8154) centre (18.7888, -0.5434) ccw
  arc A409 (18.7975, -5.8154) -> (19.1913, -5.8026) centre (18.7875, 0.5924) ccw
  arc A410 (19.1913, -5.8026) -> (19.6752, -5.7565) centre (18.7136, 1.7696) ccw
  arc A411 (18.883, -4.3384) -> (19.1958, -4.3226) centre (18.7735, 0.9324) ccw
  arc A412 (19.1958, -4.3226) -> (19.5874, -4.279) centre (18.6831, 2.0646) ccw
  arc A413 (19.5874, -4.279) -> (20.0662, -4.1951) centre (18.517, 3.2324) ccw
  arc A414 (19.1652, -2.8435) -> (19.4758, -2.8032) centre (18.6425, 2.4025) ccw
  arc A415 (19.4758, -2.8032) -> (19.8627, -2.729) centre (18.4635, 3.5241) ccw
  arc A416 (19.8627, -2.729) -> (20.3335, -2.6078) centre (18.2064, 4.6753) ccw
  arc A417 (19.3292, -1.331) -> (19.6357, -1.2665) centre (18.3965, 3.8577) ccw
  arc A418 (19.6357, -1.2665) -> (20.0156, -1.1622) centre (18.1301, 4.9618) ccw
  arc A419 (20.0156, -1.1622) -> (20.4754, -1.0044) centre (17.7834, 6.0894) ccw
  arc A420 (19.3741, 0.1896) -> (19.6745, 0.278) centre (18.0371, 5.2892) ccw
  arc A421 (19.6745, 0.278) -> (20.0451, 0.4118) centre (17.6849, 6.369) ccw
  arc A422 (20.0451, 0.4118) -> (20.4911, 0.6052) centre (17.2508, 7.4658) ccw
  arc A423 (19.2995, 1.7091) -> (19.592, 1.8208) centre (17.5665, 6.6881) ccw
  arc A424 (19.592, 1.8208) -> (19.951, 1.9832) centre (17.1307, 7.7369) ccw
  arc A425 (19.951, 1.9832) -> (20.3804, 2.2111) centre (16.6119, 8.7963) ccw
  arc A426 (19.1059, 3.2181) -> (19.3888, 3.3524) centre (16.9876, 8.0457) ccw
  arc A427 (19.3888, 3.3524) -> (19.7339, 3.5425) centre (16.4708, 9.0571) ccw
  arc A428 (19.7339, 3.5425) -> (20.1441, 3.8033) centre (15.8705, 10.0726) ccw
  arc A429 (18.7945, 4.7072) -> (19.066, 4.8632) centre (16.304, 9.3537) ccw
  arc A430 (19.066, 4.8632) -> (19.3951, 5.0799) centre (15.7095, 10.3215) ccw
  arc A431 (19.3951, 5.0799) -> (19.7836, 5.372) centre (15.0313, 11.2867) ccw
  arc A432 (18.3672, 6.1673) -> (18.6257, 6.3442) centre (15.5199, 10.6041) ccw
  arc A433 (18.6257, 6.3442) -> (18.9368, 6.5859) centre (14.8512, 11.5222) ccw
  arc A434 (18.9368, 6.5859) -> (19.3011, 6.9077) centre (14.0994, 12.4312) ccw
  arc A435 (17.8267, 7.5893) -> (18.0705, 7.786) centre (14.64, 11.7891) ccw
  arc A436 (18.0705, 7.786) -> (18.3617, 8.0514) centre (13.9014, 12.6519) ccw
  arc A437 (18.3617, 8.0514) -> (18.6997, 8.4007) centre (13.0806, 13.4991) ccw
  arc A438 (17.1763, 8.9646) -> (17.4039, 9.1797) centre (13.6699, 12.9014) ccw
  arc A439 (17.4039, 9.1797) -> (17.6718, 9.4654) centre (12.8659, 13.7036) ccw
  arc A440 (17.6718, 9.4654) -> (17.9829, 9.842) centre (11.9812, 14.4838) ccw
  arc A441 (16.42, 10.2846) -> (16.63, 10.5169) centre (12.6156, 13.9341) ccw
  arc A442 (16.63, 10.5169) -> (16.8761, 10.8246) centre (11.7511, 14.6708) ccw
  arc A443 (16.8761, 10.8246) -> (17.1553, 11.2226) centre (10.8078, 15.3792) ccw
  arc A444 (15.5625, 11.5412) -> (15.7536, 11.7893) centre (11.4834, 14.881) ccw
  arc A445 (15.7536, 11.7893) -> (15.9748, 12.1154) centre (10.5638, 15.5476) ccw
  arc A446 (15.9748, 12.1154) -> (16.2219, 12.534) centre (9.5679, 16.1798) ccw
  arc A447 (14.609, 12.7266) -> (14.7786, 12.9866) centre (10.2805, 15.7361) ccw
  arc A448 (14.7786, 12.9866) -> (14.975, 13.3314) centre (9.3114, 16.3285) ccw
  arc A449 (14.975, 13.3314) -> (15.1885, 13.7681) centre (8.2689, 16.8806) ccw
  arc A450 (13.5655, 13.8336) -> (13.7141, 14.1061) centre (9.0141, 16.4942) ccw
  arc A451 (13.7141, 14.1061) -> (13.8828, 14.4652) centre (8.0015, 17.0087) ccw
  arc A452 (13.8828, 14.4652) -> (14.0614, 14.9173) centre (6.919, 17.4773) ccw
  arc A453 (12.4383, 14.8553) -> (12.5662, 15.1412) centre (7.6922, 17.1506) ccw
  arc A454 (12.5662, 15.1412) -> (12.7051, 15.5098) centre (6.6424, 17.5841) ccw
  arc A455 (12.7051, 15.5098) -> (12.8477, 15.9746) centre (5.5264, 17.9663) ccw
  arc A456 (11.2344, 15.7854) -> (11.3395, 16.0804) centre (6.3229, 17.7012) ccw
  arc A457 (11.3395, 16.0804) -> (11.4491, 16.4589) centre (5.2423, 18.051) ccw
  arc A458 (11.4491, 16.4589) -> (11.5547, 16.9334) centre (4.0998, 18.3445) ccw
  arc A459 (9.9612, 16.6182) -> (10.0429, 16.9205) centre (4.9146, 18.1428) ccw
  arc A460 (10.0429, 16.9205) -> (10.1224, 17.3064) centre (3.8099, 18.4067) ccw
  arc A461 (10.1224, 17.3064) -> (10.1905, 17.7877) centre (2.6478, 18.6096) ccw
  arc A462 (8.6267, 17.3485) -> (8.6843, 17.6563) centre (3.476, 18.4724) ccw
  arc A463 (8.6843, 17.6563) -> (8.7334, 18.0473) centre (2.3539, 18.6488) ccw
  arc A464 (8.7334, 18.0473) -> (8.7635, 18.5324) centre (1.1796, 18.76) ccw
  arc A465 (7.2389, 17.9719) -> (7.2723, 18.2833) centre (2.0159, 18.6882) ccw
  arc A466 (7.2723, 18.2833) -> (7.2905, 18.6768) centre (0.8835, 18.776) ccw
  arc A467 (7.2905, 18.6768) -> (7.2825, 19.1629) centre (-0.2959, 18.7947) ccw
  arc A468 (5.8066, 18.4844) -> (5.8154, 18.7975) centre (0.5434, 18.7888) ccw
  arc A469 (5.8154, 18.7975) -> (5.8026, 19.1913) centre (-0.5924, 18.7875) ccw
  arc A470 (5.8026, 19.1913) -> (5.7565, 19.6752) centre (-1.7696, 18.7136) ccw
  arc A471 (4.3384, 18.883) -> (4.3226, 19.1958) centre (-0.9324, 18.7735) ccw
  arc A472 (4.3226, 19.1958) -> (4.279, 19.5874) centre (-2.0646, 18.6831) ccw
  arc A473 (4.279, 19.5874) -> (4.1951, 20.0662) centre (-3.2324, 18.517) ccw
  arc A474 (2.8435, 19.1652) -> (2.8032, 19.4758) centre (-2.4025, 18.6425) ccw
  arc A475 (2.8032, 19.4758) -> (2.729, 19.8627) centre (-3.5241, 18.4635) ccw
  arc A476 (2.729, 19.8627) -> (2.6078, 20.3335) centre (-4.6753, 18.2064) ccw
  arc A477 (1.331, 19.3292) -> (1.2665, 19.6357) centre (-3.8577, 18.3965) ccw
  arc A478 (1.2665, 19.6357) -> (1.1622, 20.0156) centre (-4.9618, 18.1301) ccw
  arc A479 (1.1622, 20.0156) -> (1.0044, 20.4754) centre (-6.0894, 17.7834) ccw
  arc A480 (0.1896, 19.3741) -> (-0.1896, 19.3741) centre (0, 0) ccw
  arc A481 (-1.331, 19.3292) -> (-1.7091, 19.2995) centre (0, 0) ccw
  arc A482 (-2.8435, 19.1652) -> (-3.2181, 19.1059) centre (0, 0) ccw
  arc A483 (-4.3384, 18.883) -> (-4.7072, 18.7945) centre (0, 0) ccw
  arc A484 (-5.8066, 18.4844) -> (-6.1673, 18.3672) centre (0, 0) ccw
  arc A485 (-7.2389, 17.9719) -> (-7.5893, 17.8267) centre (0, 0) ccw
  arc A486 (-8.6267, 17.3485) -> (-8.9646, 17.1763) centre (0, 0) ccw
  arc A487 (-9.9612, 16.6182) -> (-10.2846, 16.42) centre (0, 0) ccw
  arc A488 (-11.2344, 15.7854) -> (-11.5412, 15.5625) centre (0, 0) ccw
  arc A489 (-12.4383, 14.8553) -> (-12.7266, 14.609) centre (0, 0) ccw
  arc A490 (-13.5655, 13.8336) -> (-13.8336, 13.5655) centre (0, 0) ccw
  arc A491 (-14.609, 12.7266) -> (-14.8553, 12.4383) centre (0, 0) ccw
  arc A492 (-15.5625, 11.5412) -> (-15.7854, 11.2344) centre (0, 0) ccw
  arc A493 (-16.42, 10.2846) -> (-16.6182, 9.9612) centre (0, 0) ccw
  arc A494 (-17.1763, 8.9646) -> (-17.3485, 8.6267) centre (0, 0) ccw
  arc A495 (-17.8267, 7.5893) -> (-17.9719, 7.2389) centre (0, 0) ccw
  arc A496 (-18.3672, 6.1673) -> (-18.4844, 5.8066) centre (0, 0) ccw
  arc A497 (-18.7945, 4.7072) -> (-18.883, 4.3384) centre (0, 0) ccw
  arc A498 (-19.1059, 3.2181) -> (-19.1652, 2.8435) centre (0, 0) ccw
  arc A499 (-19.2995, 1.7091) -> (-19.3292, 1.331) centre (0, 0) ccw
  arc A500 (-19.3741, 0.1896) -> (-19.3741, -0.1896) centre (0, 0) ccw
  arc A501 (-19.3292, -1.331) -> (-19.2995, -1.7091) centre (0, 0) ccw
  arc A502 (-19.1652, -2.8435) -> (-19.1059, -3.2181) centre (0, 0) ccw
  arc A503 (-18.883, -4.3384) -> (-18.7945, -4.7072) centre (0, 0) ccw
  arc A504 (-18.4844, -5.8066) -> (-18.3672, -6.1673) centre (0, 0) ccw
  arc A505 (-17.9719, -7.2389) -> (-17.8267, -7.5893) centre (0, 0) ccw
  arc A506 (-17.3485, -8.6267) -> (-17.1763, -8.9646) centre (0, 0) ccw
  arc A507 (-16.6182, -9.9612) -> (-16.42, -10.2846) centre (0, 0) ccw
  arc A508 (-15.7854, -11.2344) -> (-15.5625, -11.5412) centre (0, 0) ccw
  arc A509 (-14.8553, -12.4383) -> (-14.609, -12.7266) centre (0, 0) ccw
  arc A510 (-13.8336, -13.5655) -> (-13.5655, -13.8336) centre (0, 0) ccw
  arc A511 (-12.7266, -14.609) -> (-12.4383, -14.8553) centre (0, 0) ccw
  arc A512 (-11.5412, -15.5625) -> (-11.2344, -15.7854) centre (0, 0) ccw
  arc A513 (-10.2846, -16.42) -> (-9.9612, -16.6182) centre (0, 0) ccw
  arc A514 (-8.9646, -17.1763) -> (-8.6267, -17.3485) centre (0, 0) ccw
  arc A515 (-7.5893, -17.8267) -> (-7.2389, -17.9719) centre (0, 0) ccw
  arc A516 (-6.1673, -18.3672) -> (-5.8066, -18.4844) centre (0, 0) ccw
  arc A517 (-4.7072, -18.7945) -> (-4.3384, -18.883) centre (0, 0) ccw
  arc A518 (-3.2181, -19.1059) -> (-2.8435, -19.1652) centre (0, 0) ccw
  arc A519 (-1.7091, -19.2995) -> (-1.331, -19.3292) centre (0, 0) ccw
  arc A520 (-0.1896, -19.3741) -> (0.1896, -19.3741) centre (0, 0) ccw
  arc A521 (1.331, -19.3292) -> (1.7091, -19.2995) centre (0, 0) ccw
  arc A522 (2.8435, -19.1652) -> (3.2181, -19.1059) centre (0, 0) ccw
  arc A523 (4.3384, -18.883) -> (4.7072, -18.7945) centre (0, 0) ccw
  arc A524 (5.8066, -18.4844) -> (6.1673, -18.3672) centre (0, 0) ccw
  arc A525 (7.2389, -17.9719) -> (7.5893, -17.8267) centre (0, 0) ccw
  arc A526 (8.6267, -17.3485) -> (8.9646, -17.1763) centre (0, 0) ccw
  arc A527 (9.9612, -16.6182) -> (10.2846, -16.42) centre (0, 0) ccw
  arc A528 (11.2344, -15.7854) -> (11.5412, -15.5625) centre (0, 0) ccw
  arc A529 (12.4383, -14.8553) -> (12.7266, -14.609) centre (0, 0) ccw
  arc A530 (13.5655, -13.8336) -> (13.8336, -13.5655) centre (0, 0) ccw
  arc A531 (14.609, -12.7266) -> (14.8553, -12.4383) centre (0, 0) ccw
  arc A532 (15.5625, -11.5412) -> (15.7854, -11.2344) centre (0, 0) ccw
  arc A533 (16.42, -10.2846) -> (16.6182, -9.9612) centre (0, 0) ccw
  arc A534 (17.1763, -8.9646) -> (17.3485, -8.6267) centre (0, 0) ccw
  arc A535 (17.8267, -7.5893) -> (17.9719, -7.2389) centre (0, 0) ccw
  arc A536 (18.3672, -6.1673) -> (18.4844, -5.8066) centre (0, 0) ccw
  arc A537 (18.7945, -4.7072) -> (18.883, -4.3384) centre (0, 0) ccw
  arc A538 (19.1059, -3.2181) -> (19.1652, -2.8435) centre (0, 0) ccw
  arc A539 (19.2995, -1.7091) -> (19.3292, -1.331) centre (0, 0) ccw
  arc A540 (19.3741, -0.1896) -> (19.3741, 0.1896) centre (0, 0) ccw
  arc A541 (19.3292, 1.331) -> (19.2995, 1.7091) centre (0, 0) ccw
  arc A542 (19.1652, 2.8435) -> (19.1059, 3.2181) centre (0, 0) ccw
  arc A543 (18.883, 4.3384) -> (18.7945, 4.7072) centre (0, 0) ccw
  arc A544 (18.4844, 5.8066) -> (18.3672, 6.1673) centre (0, 0) ccw
  arc A545 (17.9719, 7.2389) -> (17.8267, 7.5893) centre (0, 0) ccw
  arc A546 (17.3485, 8.6267) -> (17.1763, 8.9646) centre (0, 0) ccw
  arc A547 (16.6182, 9.9612) -> (16.42, 10.2846) centre (0, 0) ccw
  arc A548 (15.7854, 11.2344) -> (15.5625, 11.5412) centre (0, 0) ccw
  arc A549 (14.8553, 12.4383) -> (14.609, 12.7266) centre (0, 0) ccw
  arc A550 (13.8336, 13.5655) -> (13.5655, 13.8336) centre (0, 0) ccw
  arc A551 (12.7266, 14.609) -> (12.4383, 14.8553) centre (0, 0) ccw
  arc A552 (11.5412, 15.5625) -> (11.2344, 15.7854) centre (0, 0) ccw
  arc A553 (10.2846, 16.42) -> (9.9612, 16.6182) centre (0, 0) ccw
  arc A554 (8.9646, 17.1763) -> (8.6267, 17.3485) centre (0, 0) ccw
  arc A555 (7.5893, 17.8267) -> (7.2389, 17.9719) centre (0, 0) ccw
  arc A556 (6.1673, 18.3672) -> (5.8066, 18.4844) centre (0, 0) ccw
  arc A557 (4.7072, 18.7945) -> (4.3384, 18.883) centre (0, 0) ccw
  arc A558 (3.2181, 19.1059) -> (2.8435, 19.1652) centre (0, 0) ccw
  arc A559 (1.7091, 19.2995) -> (1.331, 19.3292) centre (0, 0) ccw
  arc A560 (-0.6052, 20.4911) -> (-1.0044, 20.4754) centre (0, 0) ccw
  arc A561 (-2.2111, 20.3804) -> (-2.6078, 20.3335) centre (0, 0) ccw
  arc A562 (-3.8033, 20.1441) -> (-4.1951, 20.0662) centre (0, 0) ccw
  arc A563 (-5.372, 19.7836) -> (-5.7565, 19.6752) centre (0, 0) ccw
  arc A564 (-6.9077, 19.3011) -> (-7.2825, 19.1629) centre (0, 0) ccw
  arc A565 (-8.4007, 18.6997) -> (-8.7635, 18.5324) centre (0, 0) ccw
  arc A566 (-9.842, 17.9829) -> (-10.1905, 17.7877) centre (0, 0) ccw
  arc A567 (-11.2226, 17.1553) -> (-11.5547, 16.9334) centre (0, 0) ccw
  arc A568 (-12.534, 16.2219) -> (-12.8477, 15.9746) centre (0, 0) ccw
  arc A569 (-13.7681, 15.1885) -> (-14.0614, 14.9173) centre (0, 0) ccw
  arc A570 (-14.9173, 14.0614) -> (-15.1885, 13.7681) centre (0, 0) ccw
  arc A571 (-15.9746, 12.8477) -> (-16.2219, 12.534) centre (0, 0) ccw
  arc A572 (-16.9334, 11.5547) -> (-17.1553, 11.2226) centre (0, 0) ccw
  arc A573 (-17.7877, 10.1905) -> (-17.9829, 9.842) centre (0, 0) ccw
  arc A574 (-18.5324, 8.7635) -> (-18.6997, 8.4007) centre (0, 0) ccw
  arc A575 (-19.1629, 7.2825) -> (-19.3011, 6.9077) centre (0, 0) ccw
  arc A576 (-19.6752, 5.7565) -> (-19.7836, 5.372) centre (0, 0) ccw
  arc A577 (-20.0662, 4.1951) -> (-20.1441, 3.8033) centre (0, 0) ccw
  arc A578 (-20.3335, 2.6078) -> (-20.3804, 2.2111) centre (0, 0) ccw
  arc A579 (-20.4754, 1.0044) -> (-20.4911, 0.6052) centre (0, 0) ccw
  arc A580 (-20.4911, -0.6052) -> (-20.4754, -1.0044) centre (0, 0) ccw
  arc A581 (-20.3804, -2.2111) -> (-20.3335, -2.6078) centre (0, 0) ccw